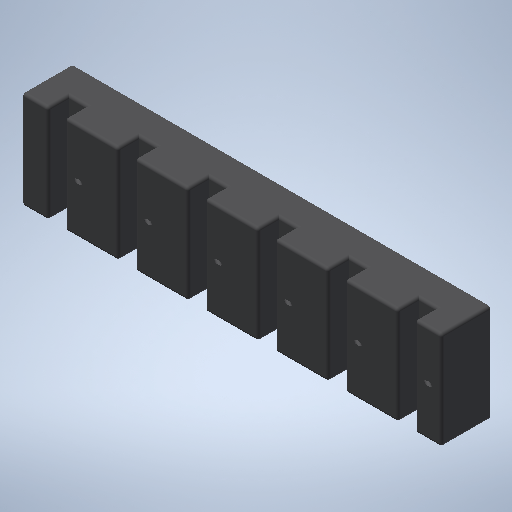
# Autodesk Inventor part: Probe Holder New_V1
Saved by Autodesk Inventor 2025.2 (Build 292293000, 293)
## iProperties
Created: 2019-02-12
Part Number: Probe Holder New_V1
Document SubType Name: Modeling
Designer: eifert
Material: Generic
Density: 1 g/cm^3
Appearance: Gray
Mass: 655.24 g
Surface Area: 778.989 cm^2
Volume: 655.24 cm^3
Author: eifert
Autodesk Inventor part; units mm, degrees
ref_plane "YZ Plane" through (0, 0, 0) normal (1, 0, 0) x (0, 1, 0)
sketch "Sketch1" plane through (0, 0, 0) normal (0, 0, 1) x (1, 0, 0)
  line L0 (-150, -35) -> (150, -35)
  line L1 (150, -35) -> (150, 35)
  line L2 (150, 35) -> (-150, 35)
  line L3 (-150, 35) -> (-150, -35)
  point P0 (0, 0)
  dimension "d0" = 300
  dimension "d1" = 70
  dimension "d57" = 150
  dimension "d58" = 35
  constraints: 8 end point, 2 parallel, 1 horizontal, 1 perpendicular
  measures "d0" distance of L0.start L0.end
  measures "d1" distance of L2.end L0.start
  measures "d57" distance from line of L3 point (0, 0)
  measures "d58" distance from line of L2 point (0, 0)
extrude "Extrusion8" add sketch "Sketch1" along normal blind 35
sketch "Sketch23" plane through (-150, 35, 0) normal (0, 1, 0) x (1, 0, 0)
  line L0 (18.95, -20) -> (31.05, -20)
  line L1 (31.05, -20) -> (31.05, -35)
  line L2 (31.05, -35) -> (18.95, -35)
  line L3 (18.95, -35) -> (18.95, -20)
  line L4 (300, -35) -> (0, -35) projected
  line L5 (0, 0) -> (0, -35) projected
  line L6 (300, 0) -> (300, -35) projected
  point P0 (150, 0)
  dimension "d175" = 15
  dimension "d176" = 12.1
  dimension "d200" = 18.95
  constraints: 8 end point, 2 parallel, 1 horizontal, 1 horizontal alignment, 1 perpendicular
  measures "d175" distance between parallel lines of L0 L4
  measures "d176" distance between parallel lines of L1 L3
  measures "d200" distance between parallel lines of L3 L5
extrude "Extrusion17" cut sketch "Sketch23" against normal through all
ref_plane "Work Plane11" through (-150, 0, 0) normal (0, 1, 0) x (1, 0, 0)
sketch "Sketch24" plane through (-150, 0, 0) normal (0, 1, 0) x (1, 0, 0)
  line L0 (18.95, -20) -> (31.05, -20) projected
  line L1 (18.95, -35) -> (18.95, -20) projected
  line L2 (31.05, -20) -> (31.05, -35) projected
  line L3 (18.95, -20) -> (18.95, -35) projected
  line L4 (18.95, -20) -> (63.1254, -50.932)
  line L5 (300, 0) -> (300, -35) projected
  point P0 (150, 0)
  dimension "d180" = 55
  constraints: 2 end point
  measures "d180" angle of L4 L5
ref_plane "Work Plane12" through (-86.8746, 0, 50.932) normal (0.819152, 0, 0.5735764) x (0, 1, 0)
sketch "Sketch25" plane through (-86.8746, 0, 50.932) normal (0.819152, 0, 0.5735764) x (0, 1, 0)
  line L0 (35, 0) -> (-35, 0) projected
  circle A0 centre (0, 0) radius 1.6
  point P0 (0, -91.5502)
  dimension "d181" = 3.2
  constraints: 1 centre point, 1 midpoint
  measures "d181" diameter of A0
extrude "Extrusion18" cut sketch "Sketch25" against normal blind 50
sketch "Sketch27" plane through (0, 0, 0) normal (0, 0, -1) x (-1, 0, 0)
  circle A0 centre (-125, 0) radius 2.5
  circle A1 centre (125, 0) radius 2.5
  circle A2 centre (0, 0) radius 2.5
  dimension "d188" = 5
  dimension "d189" = 5
  dimension "d204" = 250
  dimension "d205" = 125
  dimension "d206" = 5
  constraints: 3 centre point, 2 coincident, 2 horizontal alignment
  measures "d188" diameter of A0
  measures "d189" diameter of A1
  measures "d204" distance of A1.centre A0.centre
  measures "d205" distance of A0.centre point (0, 0)
  measures "d206" diameter of A2
extrude "Extrusion20" cut sketch "Sketch27" against normal blind 15
sketch "Sketch28" plane through (0, 0, 0) normal (0, 0, -1) x (-1, 0, 0)
  circle A0 centre (-125, 0) radius 2.5 projected
  circle A1 centre (-125, 0) radius 3.125
  circle A2 centre (125, 0) radius 2.5 projected
  circle A3 centre (125, 0) radius 3.125
  circle A4 centre (0, 0) radius 2.5 projected
  circle A5 centre (0, 0) radius 3.125
  dimension "d194" = 6.25
  dimension "d195" = 6.25
  dimension "d210" = 6.25
  constraints: 3 centre point, 3 coincident
  measures "d194" diameter of A1
  measures "d195" diameter of A3
  measures "d210" diameter of A5
extrude "Extrusion21" cut sketch "Sketch28" against normal blind 10 contours A0 | A1 | A2 | A3 | A4 | A5
pattern_linear "Rectangular Pattern5" count 6 spacing 50 along (1, 0, 0) of "Extrusion17", "Extrusion18"
fillet "Fillet6" radius 2 68 edges at (-150, 35, 17.5) (-140.525, 35, 35) (-131.05, 35, 27.5) (-125, 35, 20) (-118.95, 35, 27.5) (-50, 35, 35) (0, 35, 35) (150, 35, 17.5) (150, 0, 35) (140.525, 35, 35) (100, 35, 35) (50, 35, 35) (-100, 35, 35) (-81.05, 35, 27.5) (-75, 35, 20) (-68.95, 35, 27.5) (-31.05, 35, 27.5) (-25, 35, 20) (-18.95, 35, 27.5) (18.95, 35, 27.5) (25, 35, 20) (31.05, 35, 27.5) (68.95, 35, 27.5) (75, 35, 20) (81.05, 35, 27.5) (118.95, 35, 27.5) (125, 35, 20) (131.05, 35, 27.5) (-150, 0, 35) (-140.525, -35, 35) (-100, -35, 35) (-50, -35, 35) (0, -35, 35) (50, -35, 35) (100, -35, 35) (140.525, -35, 35) (150, -35, 17.5) (-150, -35, 17.5) (-131.05, -35, 27.5) (-125, -35, 20) (-118.95, -35, 27.5) (-81.05, -35, 27.5) (-75, -35, 20) (-68.95, -35, 27.5) (-31.05, -35, 27.5) (-25, -35, 20) (-18.95, -35, 27.5) (18.95, -35, 27.5) (25, -35, 20) (31.05, -35, 27.5) (68.95, -35, 27.5) (75, -35, 20) (81.05, -35, 27.5) (118.95, -35, 27.5) (125, -35, 20) (131.05, -35, 27.5) (131.05, 0, 35) (118.95, 0, 35) (81.05, 0, 35) (68.95, 0, 35) (31.05, 0, 35) (18.95, 0, 35) (-18.95, 0, 35) (-31.05, 0, 35) (-68.95, 0, 35) (-81.05, 0, 35) (-131.05, 0, 35) (-118.95, 0, 35)
equation "\"d57\" = 0.5 * d0"
equation "\"d58\" = 0.5 * d1"
equation "\"d188\" = d206"
equation "\"d189\" = d206"
equation "\"d205\" = 0.5 * d204"
equation "\"d86\" = 0.5 * d85"
equation "\"d85\" = 30"
body "Solid1"
